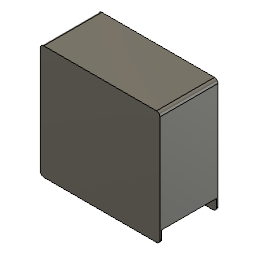
Altruist_Urban (Autodesk Fusion 360 design; units mm, degrees)
part number: 2026-10-02-14-56-16-813
part number: 2026-10-02-15-19-36-052
Autodesk Fusion 360 part; units mm, degrees
note: some values were not read from the file. Set by a fixed rule: which face or edge a step refers to.
sketch "Sketch1" plane through (0, 0, 0) normal (1, 0, 0) x (0, 0, -1) in component "Housing"
  line L0 (-51.5, 44) -> (51.5, 44)
  line L1 (51.5, 44) -> (51.5, -44)
  line L2 (51.5, -44) -> (-51.5, -44)
  line L3 (-51.5, -44) -> (-51.5, 44)
  line L4 (-51.5, 44) -> (51.5, -44) construction
  line L5 (51.5, 44) -> (-51.5, -44) construction
  dimension "d8" = 103
  dimension "d9" = 88
  constraint horizontal L0
  constraint perpendicular L0 L1
  constraint parallel L0 L2
  constraint parallel L1 L3
  constraint coincident L4 origin
  constraint coincident L5 origin
  measures "d8" distance of L0.start L0.end
  measures "d9" distance of L0.start L2.end
sketch "Sketch2" plane through (0, 0, 0) normal (0, 0, 1) x (1, 0, 0) in component "Housing"
  line L0 (-51.5, 44) -> (51.5, 44)
  line L1 (51.5, 44) -> (51.5, -44)
  line L2 (51.5, -44) -> (-51.5, -44)
  line L3 (-51.5, -44) -> (-51.5, 44)
  line L4 (-51.5, 44) -> (51.5, -44) construction
  line L5 (51.5, 44) -> (-51.5, -44) construction
  dimension "d14" = 103
  dimension "d15" = 88
  constraint horizontal L0
  constraint perpendicular L0 L1
  constraint parallel L0 L2
  constraint parallel L1 L3
  constraint coincident L4 origin
  constraint coincident L5 origin
  measures "d14" distance of L0.start L0.end
  measures "d15" distance of L0.start L2.end
extrude "Extrude2" add sketch "Sketch2" along normal blind 50 in component "Housing"
fillet "Fillet2" radius 3 2 edges at (-51.5, 44, 25) (51.5, 44, 25) in component "Housing"
shell "Shell1" thickness 3 removed faces 1 at (17.1667, -44, 16.6667) in component "Housing"
ref_plane "WorkPlane1" through (0, -38.5, 25) normal (0, -1, 0) x (1, 0, 0) in component "Housing"
split_face "SplitFace1" 4 faces at (-16.1667, 12.6667, 3) (48.5, 12.6667, 32.3333) (-16.1667, 12.6667, 47) (-48.5, -15.6667, 32.3333) by plane through (0, -38.5, 25) normal (0, -1, 0) in component "Housing"
move_face "OffsetFaces1" offset -1.6 4 faces at (16.1667, -40.3333, 3) (-48.5, -42.1667, 32.3333) (16.1667, -40.3333, 47) (48.5, -40.3333, 17.6667) in component "Housing"
ref_plane "WorkPlane3" through (0, -41.25, 25) normal (0, 0, 1) x (1, 0, 0) in component "Housing"
sketch "Sketch3 Sife Latch" plane through (0, 0, 25) normal (0, 0, 1) x (1, 0, 0) in component "Housing"
  line L0 (50.1, -42) -> (50.1, -41)
  line L1 (50.1, -41) -> (49.5, -41)
  line L2 (49.5, -41) -> (50.1, -42)
  line L3 (50.1, -38.5) -> (50.1, -44)
  dimension "d27" = 1
  dimension "d28" = 0.6
  dimension "d29" = 2
  constraint vertical L0
  constraint perpendicular L0 L1
  constraint coincident L0.start L3
  measures "d27" distance of L0.start L0.end
  measures "d28" distance of L0.end L1.end
  measures "d29" distance of L0.start L3.end
extrude "Extrude3" add sketch "Sketch3 Sife Latch" along normal mid plane 38.8 in component "Housing"
ref_plane "WorkPlane4" through (0, -41.25, 25) normal (-1, 0, 0) x (0, -1, 0) in component "Housing"
mirror "Mirror1" about plane through (0, -41.25, 25) normal (-1, 0, 0) of "Extrude3" in component "Housing"
ref_plane "WorkPlane5" through (25.05, -41.25, 25) normal (-1, 0, 0) x (0, -1, 0) in component "Housing"
sketch "Sketch4" plane through (25.05, 0, 0) normal (-1, 0, 0) x (0, 0, 1) in component "Housing"
  line L0 (1.4, -42) -> (1.4, -41)
  line L1 (1.4, -41) -> (2, -41)
  line L2 (2, -41) -> (1.4, -42)
  line L3 (1.4, -44) -> (1.4, -38.5)
  dimension "d38" = 0.6
  dimension "d39" = 1
  dimension "d40" = 2
  constraint vertical L0
  constraint perpendicular L0 L1
  constraint coincident L0.start L3
  measures "d38" distance of L0.end L1.end
  measures "d39" distance of L0.start L0.end
  measures "d40" distance of L0.start L3.start
extrude "Extrude4" add sketch "Sketch4" along normal mid plane 16 in component "Housing"
mirror "Mirror2" about plane through (0, -41.25, 25) normal (-1, 0, 0) of "Extrude4" in component "Housing"
mirror "Mirror3" about plane through (0, -41.25, 25) normal (0, 0, 1) of "Extrude4", "Mirror2" in component "Housing"
sketch "Sketch5" plane through (0, 41, 0) normal (0, -1, 0) x (1, 0, 0) in component "Housing"
  line L0 (-48.5, 47) -> (-48.5, 3)
  line L1 (-48.5, 3) -> (48.5, 3)
  line L2 (48.5, 3) -> (48.5, 47)
  line L3 (48.5, 47) -> (-48.5, 47)
  line L4 (-48.5, 41) -> (-44.5, 41)
  line L5 (-44.5, 41) -> (-44.5, 40)
  line L6 (-44.5, 40) -> (-48.5, 40)
  line L7 (-48.5, 40) -> (-48.5, 41)
  line L8 (-48.5, 37.8) -> (-44.5, 37.8)
  line L9 (-44.5, 37.8) -> (-44.5, 36.8)
  line L10 (-44.5, 36.8) -> (-48.5, 36.8)
  line L11 (-48.5, 36.8) -> (-48.5, 37.8)
  dimension "d52" = 4
  dimension "d53" = 1
  dimension "d54" = 4
  dimension "d55" = 1
  dimension "d56" = 2.2
  dimension "d57" = 6
  constraint horizontal L4
  constraint vertical L5
  constraint horizontal L6
  constraint vertical L7
  constraint coincident L0 L4.start
  constraint horizontal L8
  constraint vertical L9
  constraint horizontal L10
  constraint vertical L11
  constraint coincident L0 L8.start
  measures "d52" distance of L4.start L4.end
  measures "d53" distance of L4.end L5.end
  measures "d54" distance of L8.start L8.end
  measures "d55" distance of L8.end L9.end
  measures "d56" distance of L6.end L8.start
  measures "d57" distance of L0.start L4.start
extrude "Extrude5" add sketch "Sketch5" along normal blind 79.5 contours L0 L4 L5 L6 L7 | L0 L8 L9 L10 L11 in component "Housing"
ref_plane "WorkPlane6" through (0, 1.25, 38.9) normal (1, 0, 0) x (0, 1, 0) in component "Housing"
mirror "Mirror4" about plane through (0, 1.25, 38.9) normal (1, 0, 0) of "Extrude5" in component "Housing"
sketch "Sketch6" plane through (-48.5, 0, 0) normal (1, 0, 0) x (0, 0, -1) in component "Housing"
  line L0 (-37.8, -38.5) -> (-37.8, 41)
  line L1 (-37.8, 41) -> (-40, 41)
  line L2 (-40, 41) -> (-40, -38.5)
  line L3 (-40, -38.5) -> (-37.8, -38.5)
  line L4 (-37.8, -33.5) -> (-40, -33.5)
  line L5 (-40, -33.5) -> (-40, -32.5)
  line L6 (-40, -32.5) -> (-37.8, -32.5)
  line L7 (-37.8, -32.5) -> (-37.8, -33.5)
  line L8 (-37.8, -33) -> (-40, -33)
  dimension "d65" = 2.2
  dimension "d66" = 1
  dimension "d67" = 5
  constraint horizontal L4
  constraint vertical L5
  constraint horizontal L6
  constraint vertical L7
  constraint coincident L0 L4.start
  constraint midpoint L7 L8.start
  constraint midpoint L5 L8.end
  measures "d65" distance of L4.start L4.end
  measures "d66" distance of L4.start L6.end
  measures "d67" distance of L2.end L4.end
revolve "Revolve1" cut sketch "Sketch6" angle 180 about axis through (-48.5, -33, 37.8) along (0, 0, 1) second angle 180 contours L0 L2 L4 L5 L7 L8 in component "Housing"
mirror "Mirror5" about plane through (0, 1.25, 38.9) normal (1, 0, 0) of "Revolve1" in component "Housing"
sketch "Sketch7" plane through (0, -44, 0) normal (0, -1, 0) x (1, 0, 0) in component "Housing"
  line L0 (50.1, 48.6) -> (50.1, 1.4)
  line L1 (50.1, 1.4) -> (-50.1, 1.4)
  line L2 (-50.1, 1.4) -> (-50.1, 48.6)
  line L3 (-50.1, 48.6) -> (50.1, 48.6)
  line L4 (-51.5, 0) -> (51.5, 0)
  line L5 (51.5, 0) -> (51.5, 50)
  line L6 (51.5, 50) -> (-51.5, 50)
  line L7 (-51.5, 50) -> (-51.5, 0)
  line L8 (-51.5, 50) -> (51.5, 50)
  line L9 (51.5, 50) -> (51.5, 48.6)
  line L10 (51.5, 48.6) -> (-51.5, 48.6)
  line L11 (-51.5, 48.6) -> (-51.5, 50)
  dimension "d75" = 103
  dimension "d76" = 1.4
  constraint horizontal L8
  constraint vertical L9
  constraint horizontal L10
  constraint vertical L11
  constraint coincident L6.end L7.start
  measures "d75" distance of L6.end L5.end
  measures "d76" distance of L6.end L10.end
extrude "Extrude6" add sketch "Sketch7" along normal blind 10 contours L3 L5 L6 L7 L8 L9 L10 L11 in component "Housing"
fillet "Fillet3" radius 3 2 edges at (-51.5, -54, 49.3) (51.5, -54, 49.3) in component "Housing"
mirror "Mirror6" about plane through (0, -41.25, 25) normal (0, 0, 1) of "Extrude6", "Fillet3" in component "Housing"
component "Housing" placed x (1, 0, 0) y (0, 1, 0) z (0, 0, 1) at (0, 0, 0)
equation "HousingWidth = 103 mm"
equation "HousingHeight = 88 mm"
equation "HousingDepth = 50 mm"
equation "HousingCornerRadius = 3 mm"
equation "HousingWallThickness = 3 mm"
equation "d8 = HousingWidth"
equation "d9 = HousingHeight"
equation "d14 = HousingWidth"
equation "d15 = HousingHeight"
equation "d16 = HousingDepth"
equation "d19 = HousingCornerRadius"
equation "d20 = HousingWallThickness"
equation "HousingClosingGap = 5.5 mm"
equation "d22 = -HousingClosingGap"
equation "d24 = -HousingWallThickness / 2 - 0.1 mm"
equation "HousingLatchHeight = 1 mm"
equation "HousingLatchWidth = 0.6 mm"
equation "d27 = HousingLatchHeight"
equation "d28 = HousingLatchWidth"
equation "d29 = HousingLatchBottom"
equation "HousingLatchBottom = 2 mm"
equation "HousingLatchDepth = 38.8 mm"
equation "d33 = HousingLatchDepth / 2"
equation "HousingLatchFrontDepth = 16 mm"
equation "d38 = HousingLatchWidth"
equation "d39 = HousingLatchHeight"
equation "d40 = HousingLatchBottom"
equation "d41 = HousingLatchFrontDepth / 2"
equation "HousingRailThickness = 1 mm"
equation "HousingRailsHeight = HousingHeight - HousingClosingGap - HousingWallThickness"
equation "HousingRailWidth = 4 mm"
equation "HousingRailsOffset = 2.2 mm"
equation "HousingRailsOffsetFromFront = 6 mm"
equation "d52 = HousingRailWidth"
equation "d53 = HousingRailThickness"
equation "d54 = HousingRailWidth"
equation "d55 = HousingRailThickness"
equation "d56 = HousingRailsOffset"
equation "d57 = HousingRailsOffsetFromFront"
equation "d58 = HousingRailsHeight"
equation "HousingGrooveWidth = HousingRailsOffset"
equation "HousingGrooveHeight = 1 mm"
equation "HousingGrooveOffset = 5 mm"
equation "d65 = HousingGrooveWidth"
equation "d66 = HousingGrooveHeight"
equation "d67 = HousingGrooveOffset"
equation "HousingSkirtThickness = HousingWallThickness / 2 - 0.1 mm"
equation "HousingSkirtHeight = 10 mm"
equation "HousingSkirtWidth = HousingWidth"
equation "d75 = HousingSkirtWidth"
equation "d76 = HousingSkirtThickness"
equation "d77 = HousingSkirtHeight"
equation "d80 = HousingCornerRadius"
